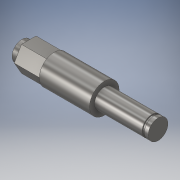
# Autodesk Inventor part: Gear - Drive Axle
Saved by Autodesk Inventor 2019.4 (Build 234330000, 330)
## iProperties
Created: 2019-11-30
Part Number: Gear - Drive Axle
Material: Steel, Mild
Document SubType Name: Modeling
Designer: admin
Density: 7.85 g/cm^3
Appearance: Semi-Polished
Mass: 72.06 g
Surface Area: 31.5463 cm^2
Volume: 9.17962 cm^3
Author: admin
Autodesk Inventor part; units mm, degrees
ref_plane "YZ Plane" through (0, 0, 0) normal (1, 0, 0) x (0, 1, 0)
ref_plane "XZ Plane" through (0, 0, 0) normal (0, 1, 0) x (-1, 0, 0)
ref_plane "XY Plane" through (0, 0, 0) normal (0, 0, 1) x (1, 0, 0)
sketch "Sketch1" plane through (0, 0, 0) normal (0, 0, 1) x (1, 0, 0)
  line L0 (0, 0) -> (0, 5)
  line L1 (0, 5) -> (3.5, 5)
  line L2 (3.5, 5) -> (3.5, 7.5)
  line L3 (3.5, 7.5) -> (41.85, 7.5)
  line L4 (41.85, 7.5) -> (41.85, 5)
  line L5 (41.85, 5) -> (66.05, 5)
  line L6 (66.05, 5) -> (66.05, 4.5)
  line L7 (66.05, 4.5) -> (67.15, 4.5)
  line L8 (67.15, 4.5) -> (67.15, 5)
  line L9 (67.15, 5) -> (69.15, 5)
  line L10 (69.15, 5) -> (69.15, 0)
  line L11 (69.15, 0) -> (0, 0)
  dimension "d0" = 5
  dimension "d1" = 7.5
  dimension "d2" = 5
  dimension "d3" = 1.1
  dimension "d4" = 0.5
  dimension "d5" = 62.55
  dimension "d6" = 2
  dimension "d7" = 3.5
  dimension "d8" = 38.35
  constraints: 24 end point, 9 perpendicular, 2 point on line, 2 vertical
  measures "d0" distance between parallel lines of L11 L1
  measures "d1" distance between parallel lines of L11 L3
  measures "d2" distance between parallel lines of L11 L5
  measures "d3" distance of L6.end L7.end
  measures "d4" distance of L5.end L6.end
  measures "d5" distance between parallel lines of L6 L2
  measures "d6" distance of L8.end L9.end
  measures "d7" distance of L0.end L1.end
  measures "d8" distance of L2.end L3.end
revolve "Revolution1" add sketch "Sketch1" angle 360 about axis through (69.15, 0, 0) along (-1, 0, 0)
sketch "Sketch2" plane through (3.5, 0, 0) normal (-1, 0, 0) x (0, 0, 1)
  line L0 (3.7107, 6.3753) -> (7.3765, -0.0259)
  line L1 (7.3765, -0.0259) -> (3.6658, -6.4012)
  line L2 (3.6658, -6.4012) -> (-3.7107, -6.3753)
  line L3 (-3.7107, -6.3753) -> (-7.3765, 0.0259)
  line L4 (-7.3765, 0.0259) -> (-3.6658, 6.4012)
  line L5 (-3.6658, 6.4012) -> (3.7107, 6.3753)
  circle A0 centre (0, 0) radius 7.5 projected
  circle A1 centre (0, 0) radius 5 projected
  point P0 (0, 0)
  point P1 (0, 0)
  dimension "d10" = 14.753
  constraints: 12 end point, 1 coincident, 13 other
  measures "d10" horizontal distance of L0.end L3.end
extrude "Extrusion1" cut sketch "Sketch2" against normal blind 12.849 contours A0
body "Solid1"
